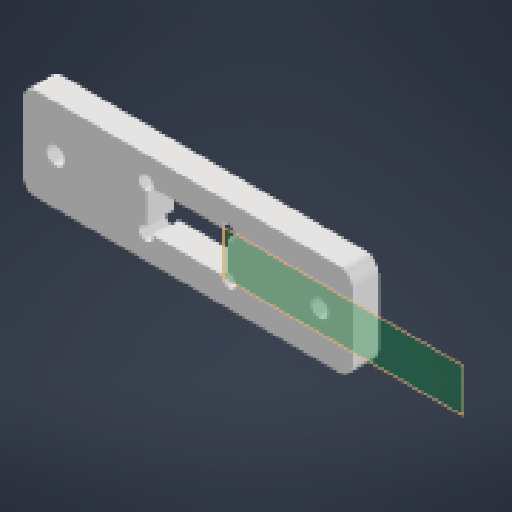
# Autodesk Inventor part: zig8
Saved by Autodesk Inventor 2024.3 (Build 283343000, 343)
## iProperties
Created: 2024-09-11
Part Number: zig8
Material: 일반
Document SubType Name: Modeling
Designer: ASUS
Density: 1 g/cm^3
Appearance: 기본값
Author: ASUS
Autodesk Inventor part; units mm, degrees
ref_plane "YZ Plane" through (0, 0, 0) normal (1, 0, 0) x (0, 1, 0)
ref_plane "XZ Plane" through (0, 0, 0) normal (0, 1, 0) x (-1, 0, 0)
ref_plane "XY Plane" through (0, 0, 0) normal (0, 0, 1) x (1, 0, 0)
ref_plane "작업 평면1" through (80.2, 0, -34) normal (0, 0, -1) x (-1, 0, 0)
sketch "스케치1" plane through (80.2, 0, -34) normal (0, 0, -1) x (-1, 0, 0)
  line L0 (34.1, 0) -> (46.1, 0) projected
  line L1 (46.1, 0) -> (46.1, 6) projected
  line L2 (34.1, 6) -> (46.1, 6) projected
  line L3 (34.1, 0) -> (34.1, 6) projected
  line L4 (46.2, 6.1) -> (46.2, -0.1)
  line L5 (46.2, -0.1) -> (34, -0.1)
  line L6 (34, -0.1) -> (34, 6.1)
  line L7 (34, 6.1) -> (46.2, 6.1)
  line L8 (33.1, 0) -> (33.1, 6) projected
  line L9 (0, 6) -> (33.1, 6) projected
  line L10 (0, 0) -> (0, 6) projected
  line L11 (0, 0) -> (33.1, 0) projected
  circle A0 centre (20.1, 3) radius 1.35 projected
  line L12 (47.1, 6) -> (47.1, 0) projected
  line L13 (47.1, 0) -> (80.2, 0) projected
  line L14 (80.2, 0) -> (80.2, 6) projected
  line L15 (47.1, 6) -> (80.2, 6) projected
  circle A1 centre (60.1, 3) radius 1.35 projected
  line L16 (50.1, 10) -> (50.1, -4)
  line L17 (50.1, -4) -> (30.1, -4)
  line L18 (30.1, -4) -> (30.1, 10)
  line L19 (30.1, 10) -> (50.1, 10)
  line L20 (15.1, -4) -> (25.1, -4)
  line L21 (25.1, -4) -> (25.1, 10)
  line L22 (25.1, 10) -> (15.1, 10)
  line L23 (15.1, 10) -> (15.1, -4)
  line L24 (15.1, -4) -> (25.1, 10) construction
  line L25 (25.1, -4) -> (15.1, 10) construction
  line L26 (55.1, -4) -> (65.1, -4)
  line L27 (65.1, -4) -> (65.1, 10)
  line L28 (65.1, 10) -> (55.1, 10)
  line L29 (55.1, 10) -> (55.1, -4)
  line L30 (55.1, -4) -> (65.1, 10) construction
  line L31 (65.1, -4) -> (55.1, 10) construction
  line L32 (15.1, 10) -> (65.1, 10)
  line L33 (65.1, 10) -> (65.1, -4)
  line L34 (65.1, -4) -> (15.1, -4)
  line L35 (15.1, -4) -> (15.1, 10)
  circle A2 centre (34, 6.1) radius 1.05
  circle A3 centre (33.8, -0.3) radius 1.05
  circle A4 centre (46.4, -0.3) radius 1.05
  circle A5 centre (46.4, 6.3) radius 1.05
  point P0 (34, 0.7308)
  point P1 (34, 5.05)
  point P2 (35.05, 6.1)
  point P3 (45.3692, 6.1)
  point P4 (46.2, 5.2692)
  point P5 (46.2, 0.7308)
  point P6 (45.3692, -0.1)
  point P7 (34.8308, -0.1)
  point P8 (50.1, -4)
  dimension "d0" = 0.1
  dimension "d1" = 4
  dimension "d2" = 10
  dimension "d3" = 14
  dimension "d4" = 10
  dimension "d5" = 14
  dimension "d6" = 2.1
  dimension "d7" = 2.1
  dimension "d8" = 2.1
  dimension "d9" = 2.1
  constraints: 48 end point, 6 parallel, 4 centre point, 4 midpoint, 3 horizontal, 3 perpendicular, 1 coincident, 6 other
  measures "d0" distance between parallel lines of L2 L7
  measures "d1" distance between parallel lines of L2 L19
  measures "d2" distance of L22.end L21.end
  measures "d3" distance of L21.end L20.end
  measures "d4" distance of L28.end L27.end
  measures "d5" distance of L27.end L26.end
  measures "d6" diameter of A2
  measures "d7" diameter of A3
  measures "d8" diameter of A4
  measures "d9" diameter of A5
extrude "돌출1" add sketch "스케치1" along normal blind 4 contours L5 A4 L13 L16 L17 L18 L11 A3 | A3 L8 A2 L6 | A3 L11 L18 L9 A2 L8 | L4 A5 L12 A4 | A2 L9 L18 L19 L16 L15 A5 L7 | L12 A5 L15 L16 L13 A4 | L18 L34 L21 L11 | L11 L21 L9 L18 | L16 L15 L29 L13 | L13 L29 L34 L16 | L21 L20 L23 L11 | L11 L23 L9 L21 | L9 L21 L32 L18 | L29 L15 L27 L13 | L13 L27 L26 L29 | L16 L32 L29 L15 | L9 L23 L22 L21 | L29 L28 L27 L15
fillet "모깎기1" radius 2 4 edges at (15.1, -4, -36) (15.1, 10, -36) (65.1, -4, -36) (65.1, 10, -36)
